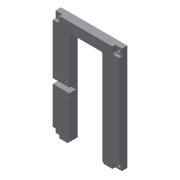
# Autodesk Inventor part: escapement base
Saved by Autodesk Inventor 2022 Beta2 (Build 260130000, 130) ContinuousBuild 0
## iProperties
Shininess: 3
Length Units: 11272
Angle Units: 11279
Time Units: 11290
Mass Units: 11286
Length Display Precision: 3
Angle Display Precision: 2
Created: 2001-07-24
Part Number: escapement base
Document SubType Name: Modeling
Designer: smithga
Density: 1 g/cm^3
Material: Generic
Appearance: Light Grey
Density: 0.0
Volumn: 0.0
Area: 0.0
PropertySet Name: Model Information
Control State: 0
Master: False
Checked Out: False
Author: smithga
Autodesk Inventor part; units mm, degrees
ref_plane "YZ Plane" through (0, 0, 0) normal (1, 0, 0) x (0, 1, 0)
ref_plane "XZ Plane" through (0, 0, 0) normal (0, 1, 0) x (-1, 0, 0)
ref_plane "XY Plane" through (0, 0, 0) normal (0, 0, 1) x (1, 0, 0)
sketch "Sketch1" plane through (0, 0, 0) normal (0, 0, 1) x (1, 0, 0)
  line L0 (127, 0) -> (127, 203.2)
  line L1 (127, 203.2) -> (0, 203.2)
  line L2 (0, 203.2) -> (0, 0)
  line L3 (95.25, 0) -> (95.25, 184.15)
  line L4 (95.25, 184.15) -> (31.75, 184.15)
  line L5 (31.75, 184.15) -> (31.75, 0)
  line L6 (0, 0) -> (31.75, 0)
  line L7 (95.25, 0) -> (127, 0)
  circle A0 centre (6.35, 6.35) radius 3.175
  circle A1 centre (120.65, 6.35) radius 3.175
  circle A2 centre (6.35, 196.85) radius 3.175
  circle A3 centre (120.65, 196.85) radius 3.175
  circle A4 centre (9.525, 101.6) radius 1.5875
  circle A5 centre (25.4, 101.6) radius 1.5875
  circle A6 centre (9.525, 76.2) radius 1.5875
  circle A7 centre (25.4, 76.2) radius 1.5875
  constraints: 16 end point, 8 centre point, 4 parallel, 2 horizontal, 2 perpendicular
extrude "Extrusion1" add sketch "Sketch1" along normal blind 15.875
chamfer "Chamfer1" distance 3.175 angle 45 2 edges at (31.75, 0, 7.9375) (95.25, 0, 7.9375)
fillet "Fillet1" radius 3.175 2 edges at (31.75, 184.15, 7.9375) (95.25, 184.15, 7.9375)
sketch "Sketch2" plane through (0, 0, 15.875) normal (0, 0, 1) x (1, 0, 0)
  arc A0 (6.35, 190.5) -> (12.7, 196.85) centre (6.35, 196.85) ccw
  line L0 (12.7, 196.85) -> (12.7, 203.2)
  line L1 (12.7, 203.2) -> (0, 203.2)
  line L2 (0, 203.2) -> (0, 190.5)
  line L3 (0, 190.5) -> (6.35, 190.5)
  arc A1 (114.3, 196.85) -> (120.65, 190.5) centre (120.65, 196.85) ccw
  line L4 (114.3, 196.85) -> (114.3, 203.2)
  line L5 (114.3, 203.2) -> (127, 203.2)
  line L6 (127, 203.2) -> (127, 190.5)
  line L7 (127, 190.5) -> (120.65, 190.5)
  arc A2 (12.7, 6.35) -> (6.35, 12.7) centre (6.35, 6.35) ccw
  line L8 (6.35, 12.7) -> (0, 12.7)
  line L9 (0, 12.7) -> (0, 0)
  line L10 (0, 0) -> (12.7, 0)
  line L11 (12.7, 0) -> (12.7, 6.35)
  arc A3 (120.65, 12.7) -> (114.3, 6.35) centre (120.65, 6.35) ccw
  line L12 (120.65, 12.7) -> (127, 12.7)
  line L13 (127, 12.7) -> (127, 0)
  line L14 (127, 0) -> (114.3, 0)
  line L15 (114.3, 0) -> (114.3, 6.35)
  constraints: 32 end point, 8 point on circle, 7 perpendicular, 5 tangent, 4 centre point, 4 parallel, 1 vertical
extrude "Extrusion2" cut sketch "Sketch2" against normal blind 5.5563
sketch "Sketch3" plane through (0, 0, 15.875) normal (0, 0, 1) x (1, 0, 0)
  line L0 (0, 93.6625) -> (31.75, 93.6625)
  line L1 (31.75, 93.6625) -> (31.75, 84.1375)
  line L2 (31.75, 84.1375) -> (0, 84.1375)
  line L3 (0, 84.1375) -> (0, 93.6625)
  constraints: 8 end point, 2 parallel, 1 horizontal, 1 perpendicular
extrude "Extrusion3" cut sketch "Sketch3" against normal blind 12.7
body "Solid1"
